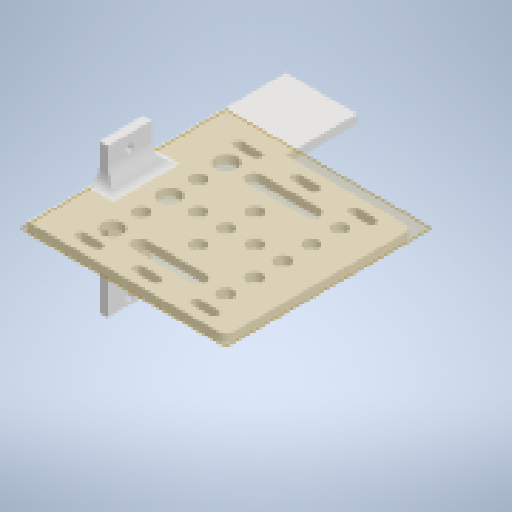
# Autodesk Inventor part: деталь основа каретки
Saved by Autodesk Inventor 2024.2 (Build 282272000, 272)
## iProperties
Created: 2026-01-31
Part Number: деталь основа каретки
Material: Типовые
Document SubType Name: Modeling
Designer: katya_notebook
Density: 1 g/cm^3
Appearance: По умолчанию
Author: katya_notebook
Autodesk Inventor part; units mm, degrees
ref_plane "YZ Plane" through (0, 0, 0) normal (1, 0, 0) x (0, 1, 0)
ref_plane "XZ Plane" through (0, 0, 0) normal (0, 1, 0) x (-1, 0, 0)
ref_plane "XY Plane" through (0, 0, 0) normal (0, 0, 1) x (1, 0, 0)
ref_plane "РабПлоскость1" through (-66.9457, 3.4254, 42.3112) normal (0, 1, 0) x (-1, 0, 0)
sketch "Эскиз1" plane through (-66.9457, 3.4254, 42.3112) normal (0, 1, 0) x (-1, 0, 0)
  arc A0 (3, 0) -> (0, 3) centre (0, 0) ccw projected
  line L0 (0, 3) -> (-59.5, 3) projected
  arc A1 (-59.5, 3) -> (-62.5, 0) centre (-59.5, 0) ccw projected
  line L1 (-62.5, 0) -> (-62.5, -59.5) projected
  arc A2 (-62.5, -59.5) -> (-59.5, -62.5) centre (-59.5, -59.5) ccw projected
  line L2 (-59.5, -62.5) -> (0, -62.5) projected
  arc A3 (0, -62.5) -> (3, -59.5) centre (0, -59.5) ccw projected
  line L3 (3, -59.5) -> (3, 0) projected
  circle A4 centre (-29.75, -29.75) radius 2.55 projected
  circle A5 centre (-39.75, -29.75) radius 2.55 projected
  circle A6 centre (-9.9, -49.75) radius 3.6 projected
  circle A7 centre (-9.9, -9.75) radius 3.6 projected
  circle A8 centre (-49.6, -49.75) radius 2.55 projected
  circle A9 centre (-49.6, -9.75) radius 2.55 projected
  circle A10 centre (-49.6, -39.75) radius 2.55 projected
  circle A11 centre (-9.9, -19.75) radius 2.55 projected
  arc A12 (-33, -55.95) -> (-33, -58.95) centre (-33, -57.45) ccw projected
  line L4 (-26.5, -55.95) -> (-33, -55.95) projected
  arc A13 (-26.5, -58.95) -> (-26.5, -55.95) centre (-26.5, -57.45) ccw projected
  line L5 (-33, -58.95) -> (-26.5, -58.95) projected
  arc A14 (-46.65, -58.95) -> (-46.65, -55.95) centre (-46.65, -57.45) ccw projected
  line L6 (-53.15, -58.95) -> (-46.65, -58.95) projected
  arc A15 (-53.15, -55.95) -> (-53.15, -58.95) centre (-53.15, -57.45) ccw projected
  line L7 (-46.65, -55.95) -> (-53.15, -55.95) projected
  arc A16 (-12.85, -0.55) -> (-12.85, -3.55) centre (-12.85, -2.05) ccw projected
  line L8 (-6.35, -0.55) -> (-12.85, -0.55) projected
  arc A17 (-6.35, -3.55) -> (-6.35, -0.55) centre (-6.35, -2.05) ccw projected
  line L9 (-12.85, -3.55) -> (-6.35, -3.55) projected
  arc A18 (-46.65, -3.55) -> (-46.65, -0.55) centre (-46.65, -2.05) ccw projected
  line L10 (-53.15, -3.55) -> (-46.65, -3.55) projected
  arc A19 (-53.15, -0.55) -> (-53.15, -3.55) centre (-53.15, -2.05) ccw projected
  line L11 (-46.65, -0.55) -> (-53.15, -0.55) projected
  arc A20 (-33, -0.55) -> (-33, -3.55) centre (-33, -2.05) ccw projected
  line L12 (-26.5, -0.55) -> (-33, -0.55) projected
  arc A21 (-26.5, -3.55) -> (-26.5, -0.55) centre (-26.5, -2.05) ccw projected
  line L13 (-33, -3.55) -> (-26.5, -3.55) projected
  arc A22 (-40.07, -7.25) -> (-40.07, -12.25) centre (-40.07, -9.75) ccw projected
  line L14 (-19.43, -7.25) -> (-40.07, -7.25) projected
  arc A23 (-19.43, -12.25) -> (-19.43, -7.25) centre (-19.43, -9.75) ccw projected
  line L15 (-40.07, -12.25) -> (-19.43, -12.25) projected
  arc A24 (-12.85, -55.95) -> (-12.85, -58.95) centre (-12.85, -57.45) ccw projected
  line L16 (-6.35, -55.95) -> (-12.85, -55.95) projected
  arc A25 (-6.35, -58.95) -> (-6.35, -55.95) centre (-6.35, -57.45) ccw projected
  line L17 (-12.85, -58.95) -> (-6.35, -58.95) projected
  arc A26 (-40.07, -47.25) -> (-40.07, -52.25) centre (-40.07, -49.75) ccw projected
  line L18 (-19.43, -47.25) -> (-40.07, -47.25) projected
  arc A27 (-19.43, -52.25) -> (-19.43, -47.25) centre (-19.43, -49.75) ccw projected
  line L19 (-40.07, -52.25) -> (-19.43, -52.25) projected
  circle A28 centre (-49.6, -19.75) radius 2.55 projected
  circle A29 centre (-29.75, -19.75) radius 2.55 projected
  circle A30 centre (-49.6, -29.75) radius 2.55 projected
  circle A31 centre (-9.9, -39.75) radius 2.55 projected
  circle A32 centre (-9.9, -29.75) radius 3.6 projected
  circle A33 centre (-19.75, -29.75) radius 2.55 projected
  circle A34 centre (-29.75, -39.75) radius 2.55 projected
  line L20 (3, -59.5) -> (3, -62.5)
  line L21 (3, -62.5) -> (0, -62.5)
  line L22 (0, 3) -> (3, 3)
  line L23 (3, 3) -> (3, 0)
  point P0 (-66.9457, -42.3112)
  constraints: 8 end point, 2 perpendicular, 1 horizontal, 1 tangent, 1 vertical
extrude "Выдавливание1" add sketch "Эскиз1" against normal blind 3
sketch "Эскиз3" plane through (-66.9457, 3.4254, 42.3112) normal (0, 1, 0) x (1, 0, 0)
  line L0 (59.5, -3) -> (-3, -3) projected
  line L1 (-3, -3) -> (-7, -3)
  line L2 (-7, -3) -> (-7, 62.5)
  line L3 (-7, 62.5) -> (-3, 62.5)
  line L4 (-3, 62.5) -> (-3, -3)
  point P0 (66.9457, 42.3112)
  dimension "d5" = 4
  constraints: 8 end point, 2 parallel, 1 horizontal, 1 perpendicular
  measures "d5" distance of L2.end L3.end
extrude "Выдавливание3" add sketch "Эскиз3" against normal blind 3
sketch "Эскиз4" plane through (-66.9457, 3.4254, 42.3112) normal (0, 1, 0) x (1, 0, 0)
  line L0 (-7, 62.5) -> (59.5, 62.5) projected
  line L1 (59.5, -3) -> (-7, -3) projected
  line L2 (-7, 62.5) -> (-4, 62.5)
  line L3 (-4, 62.5) -> (-4, -3)
  line L4 (-4, -3) -> (-7, -3)
  line L5 (-7, -3) -> (-7, 62.5)
  point P0 (66.9457, 42.3112)
  point P1 (-4, 62.5)
  dimension "d8" = 3
  constraints: 8 end point, 2 parallel, 1 horizontal, 1 perpendicular, 1 point on line
  measures "d8" distance between parallel lines of L3 L5
extrude "Выдавливание4" add sketch "Эскиз4" along normal blind 12 and the other way blind 40
sketch "Эскиз9" plane through (-66.9457, 15.4254, 42.3112) normal (0, 1, 0) x (1, 0, 0)
  line L0 (-7, 62.5) -> (-4, 62.5) projected
  line L1 (-4, 62.5) -> (-7, 62.5)
  line L2 (-7, 62.5) -> (-7, 37.5)
  line L3 (-7, 37.5) -> (-4, 37.5)
  line L4 (-4, 37.5) -> (-4, 62.5)
  line L5 (-4, -3) -> (-7, -3) projected
  line L6 (-7, 22) -> (-4, 22)
  line L7 (-4, 22) -> (-4, -3)
  line L8 (-4, -3) -> (-7, -3)
  line L9 (-7, -3) -> (-7, 22)
  point P0 (66.9457, 42.3112)
  point P1 (-7, 62.5)
  dimension "d24" = 25
  dimension "d25" = 25
  constraints: 16 end point, 4 parallel, 2 horizontal, 2 perpendicular, 1 point on line
  measures "d24" distance of L3.end L0.end
  measures "d25" distance of L6.end L5.start
extrude "Выдавливание8" cut sketch "Эскиз9" against normal blind 12
sketch "Эскиз10" plane through (-66.9457, -36.5746, 42.3112) normal (0, -1, 0) x (1, 0, 0)
  line L0 (-7, 3) -> (-7, -62.5) projected
  line L1 (-4, -37.5) -> (-7, -37.5) projected
  line L2 (-7, -62.5) -> (-4, -62.5)
  line L3 (-4, -62.5) -> (-4, -37.5)
  line L4 (-4, -37.5) -> (-7, -37.5)
  line L5 (-7, -37.5) -> (-7, -62.5)
  line L6 (-7, -22) -> (-4, -22) projected
  line L7 (-7, 3) -> (-4, 3)
  line L8 (-4, 3) -> (-4, -22)
  line L9 (-4, -22) -> (-7, -22)
  line L10 (-7, -22) -> (-7, 3)
  point P0 (66.9457, -42.3112)
  point P1 (-7, 2.6439)
  constraints: 16 end point, 4 parallel, 2 horizontal, 2 perpendicular, 2 point on line
extrude "Выдавливание9" cut sketch "Эскиз10" against normal blind 37
fillet "Сопряжение4" radius 4 4 edges at (-72.4457, 3.4254, 4.8112) (-72.4457, 0.4254, 4.8112) (-72.4457, 3.4254, 20.3112) (-72.4457, 0.4254, 20.3112)
fillet "Сопряжение5" radius 6 6 edges at (-70.9457, 3.4254, 2.8112) (-70.9457, 3.4254, 12.5612) (-70.9457, 3.4254, 22.3112) (-70.9457, 0.4254, 22.3112) (-70.9457, 0.4254, 12.5612) (-70.9457, 0.4254, 2.8112)
sketch "Эскиз11" plane through (-73.9457, -36.5746, 45.3112) normal (-1, 0, 0) x (0, 0, 1)
  circle A0 centre (-32.75, 47.5) radius 1.2 projected
  circle A1 centre (-32.75, 32.5) radius 1.2 projected
  circle A2 centre (-32.75, 17.5) radius 1.2 projected
  circle A3 centre (-32.75, 2.5) radius 1.2 projected
  point P0 (-45.3112, 36.5746)
extrude "Выдавливание10" cut sketch "Эскиз11" against normal blind 37
sketch "Эскиз12" plane through (-7.4457, 0.4254, -20.1888) normal (0, 0, -1) x (-1, 0, 0)
  line L0 (0, 0) -> (66.5, 0) projected
  line L1 (66.5, 3) -> (0, 3) projected
  line L2 (66.5, 0) -> (41.5, 0)
  line L3 (41.5, 0) -> (41.5, 3)
  line L4 (41.5, 3) -> (66.5, 3)
  line L5 (66.5, 3) -> (66.5, 0)
  point P0 (-7.4457, -0.4254)
  point P1 (41.5, 0)
  dimension "d36" = 25
  constraints: 8 end point, 2 parallel, 1 horizontal, 1 perpendicular, 1 point on line
  measures "d36" distance of L1.start L3.end
extrude "Выдавливание11" add sketch "Эскиз12" along normal blind 25
fillet "Сопряжение6" radius 6 1 edges at (-48.9457, 1.9254, -20.1888)
sketch "Эскиз13" plane through (-66.9457, 3.4254, 42.3112) normal (0, 1, 0) x (1, 0, 0)
  line L0 (15, 82.5) -> (-6.85, 82.5) projected
  line L1 (15, 59.5) -> (-6.85, 59.5) projected
  line L2 (15, 59.5) -> (15, 82.5) projected
  line L3 (-6.85, 82.5) -> (-6.85, 86) projected
  line L4 (-6.85, 56) -> (-6.85, 59.5) projected
  line L5 (18, 87.5) -> (-7, 87.5) projected
  line L6 (-6.85, 82.5) -> (15, 82.5)
  line L7 (15, 82.5) -> (15, 87.5)
  line L8 (15, 87.5) -> (-6.85, 87.5)
  line L9 (-6.85, 87.5) -> (-6.85, 82.5)
  line L10 (-6.85, 59.5) -> (15, 59.5)
  line L11 (15, 59.5) -> (15, 54.5)
  line L12 (15, 54.5) -> (-6.85, 54.5)
  line L13 (-6.85, 54.5) -> (-6.85, 59.5)
  point P0 (66.9457, 42.3112)
  point P1 (-6.85, 87.5)
  point P2 (-6.85, 86)
  point P3 (15, 82.5)
  point P4 (15, 59.5)
  dimension "d38" = 5
  constraints: 16 end point, 4 parallel, 2 horizontal, 2 perpendicular, 2 point on line
  measures "d38" distance of L10.end L11.end
extrude "Выдавливание12" add sketch "Эскиз13" along normal blind 11
sketch "Эскиз14" plane through (-73.7957, 3.4254, -45.1888) normal (-1, 0, 0) x (0, 0, 1)
  circle A0 centre (2.75, 9.5) radius 1.25 projected
  circle A1 centre (2.75, 2.5) radius 1.25 projected
  circle A2 centre (30.25, 9.5) radius 1.25 projected
  circle A3 centre (30.25, 2.5) radius 1.25 projected
  point P0 (45.1888, -3.4254)
extrude "Выдавливание13" cut sketch "Эскиз14" against normal blind 43.25
sketch "Эскиз15" plane through (-73.7957, 3.4254, -12.1888) normal (0, 0, 1) x (1, 0, 0)
  line L0 (16.35, 8.75) -> (16.35, 3.25) projected
  line L1 (0, 0) -> (0, 12) projected
  line L2 (21.85, 0) -> (0, 0) projected
  line L3 (21.85, 0) -> (21.85, 12) projected
  line L4 (21.85, 12) -> (0, 12) projected
  line L5 (16.35, 8.75) -> (13.35, 8.75) projected
  line L6 (16.35, 3.25) -> (16.35, 8.75) projected
  line L7 (13.35, 3.25) -> (16.35, 3.25) projected
  line L8 (13.35, 8.75) -> (13.35, 3.25) projected
  line L9 (13.35, 8.75) -> (16.35, 8.75)
  line L10 (16.35, 8.75) -> (16.35, 3.25)
  line L11 (16.35, 3.25) -> (13.35, 3.25)
  line L12 (13.35, 3.25) -> (13.35, 8.75)
  point P0 (73.7957, -3.4254)
  constraints: 8 end point, 2 parallel, 1 horizontal, 1 perpendicular
extrude "Выдавливание14" cut sketch "Эскиз15" against normal blind 15.75 contours L0 L7 L8 L5
sketch "Эскиз16" plane through (-73.7957, 3.4254, -12.1888) normal (0, 0, 1) x (1, 0, 0)
  line L0 (13.35, 8.25) -> (13.35, 8.75) projected
  line L1 (21.85, 0) -> (21.85, 11) projected
  line L2 (21.85, 8.75) -> (21.85, 0)
  line L3 (21.85, 0) -> (13.35, 0)
  line L4 (13.35, 0) -> (13.35, 8.75)
  line L5 (21.85, 11) -> (0, 11) projected
  line L6 (21.85, 8.75) -> (21.85, 11)
  line L7 (21.85, 11) -> (13.35, 11)
  line L8 (13.35, 11) -> (13.35, 8.75)
  point P0 (73.7957, -3.4254)
  point P1 (13.35, 11)
  constraints: 12 end point, 2 parallel
extrude "Выдавливание15" cut sketch "Эскиз16" against normal blind 15.75
fillet "Сопряжение7" radius 2 1 edges at (-67.1207, 3.4254, -12.1888)
fillet "Сопряжение8" radius 2 8 edges at (-51.9457, 3.4254, -42.6888) (-48.9457, 1.9254, -45.1888) (-73.9457, 1.9254, -45.1888) (-73.9457, 1.9254, 45.3112) (-72.4457, 15.4254, 20.3112) (-72.4457, 15.4254, 4.8112) (-72.4457, -36.5746, 4.8112) (-72.4457, -36.5746, 20.3112)
